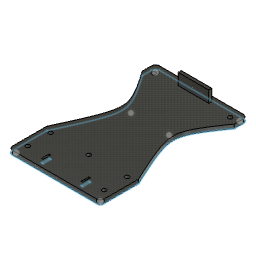
Bracket for Square Pole Mount v2 (Autodesk Fusion 360 design; units mm, degrees)
Autodesk Fusion 360 part; units mm, degrees
sketch "Sketch1" plane through (0, 0, 0) normal (0, 0, 1) x (1, 0, 0)
  line L0 (59.9937, -49.9545) -> (59.9937, -95)
  line L1 (54.9937, -100) -> (-55, -100)
  line L2 (-60, -95) -> (-60, -50)
  line L3 (-25, -90) -> (-27, -90)
  line L4 (-27, -90) -> (-27, -80)
  line L5 (-27, -80) -> (-25, -80)
  line L6 (-25, -80) -> (-25, -90)
  line L7 (25, -90) -> (27, -90)
  line L8 (27, -90) -> (27, -80)
  line L9 (27, -80) -> (25, -80)
  line L10 (25, -80) -> (25, -90)
  arc A0 (54.9937, -100) -> (59.9937, -95) centre (54.9937, -95) ccw
  arc A1 (-60, -95) -> (-55, -100) centre (-55, -95) ccw
  line L11 (-54.9833, 92.1493) -> (55.24, 92.1493)
  arc A2 (-54.9833, 92.1493) -> (-59.9833, 87.1495) centre (-54.9833, 87.1493) ccw
  arc A3 (60.24, 87.1413) -> (55.24, 92.1493) centre (55.24, 87.1493) ccw
  line L12 (-59.9833, 87.1495) -> (-59.9833, 75)
  line L13 (60.24, 87.1413) -> (60.24, 75)
  spline S0 degree 2 poles (-60, -50) (-25, 25) (-59.9833, 75) knots 0 0 0 13.576919 13.576919 13.576919 weights 1 3 1
  spline S1 degree 2 poles (59.9937, -49.9545) (25, 25) (60.24, 75) knots 0 0 0 13.58139 13.58139 13.58139 weights 1 3 1
  dimension "d78" = 5
  dimension "d79" = 5
  dimension "d98" = 5
  dimension "d99" = 5
  constraint vertical L0
  constraint horizontal L1
  constraint vertical L2
  constraint horizontal L3
  constraint vertical L4
  constraint horizontal L5
  constraint vertical L6
  constraint horizontal L7
  constraint vertical L8
  constraint horizontal L9
  constraint vertical L10
  constraint tangent L0 A0
  constraint tangent L1 A0
  constraint tangent L1 A1
  constraint tangent L2 A1
  constraint horizontal L11
  constraint tangent L11 A2
  constraint tangent L11 A3
  constraint vertical L12
  constraint vertical L13
  measures "d78" radius of A0
  measures "d79" radius of A1
  measures "d98" radius of A2
  measures "d99" radius of A3
extrude "Extrude1" add sketch "Sketch1" along normal blind 5 makes body 1
hole "Hole1" at (-50, 80, 5) direction (0, 0, -1) diameter 5.3 depth 10 tip angle 180 bodies 1
hole "Hole2" at (49.9937, 80, 5) direction (0, 0, -1) diameter 5.3 depth 10 tip angle 180 bodies 1
hole "Hole3" at (-50, -55, 5) direction (0, 0, -1) diameter 5.3 depth 10 tip angle 180 bodies 1
hole "Hole4" at (49.9937, -55, 5) direction (0, 0, -1) diameter 5.3 depth 10 tip angle 180 bodies 1
hole "Hole5" at (-50, -85, 5) direction (0, 0, -1) diameter 5.3 depth 10 tip angle 180 bodies 1
hole "Hole6" at (49.9937, -85, 5) direction (0, 0, -1) diameter 5.3 depth 10 tip angle 180 bodies 1
sketch "Sketch5" plane through (0, 0, 0) normal (0, 0, 1) x (1, 0, 0)
  line L0 (-20, 110) -> (20, 110)
  line L1 (20, 110) -> (20, 114)
  line L2 (20, 114) -> (-20, 114)
  line L3 (-20, 114) -> (-20, 110)
  constraint horizontal L0
  constraint vertical L1
  constraint horizontal L2
  constraint vertical L3
extrude "Extrude5" add sketch "Sketch5" along normal blind 20 separate body makes body 2
move_body "Move2" bodies 2 to x (1, 0, 0) y (0, 1, 0) z (0, 0, 1) at (0, -28, 0)
sketch "Sketch7" plane through (0, 0, 0) normal (1, 0, 0) x (0, 1, 0)
  line L0 (86, 10) -> (90, 5)
  line L1 (90, 5) -> (86, 5)
  line L2 (86, 5) -> (86, 10)
  constraint horizontal L1
  constraint perpendicular L1 L2
extrude "Extrude7" add sketch "Sketch7" along normal mid plane 30 bodies 1 2
hole "Hole17" at (0, -55, 5) direction (0, 0, -1) diameter 5.3 depth 30 tip angle 118 bodies 1
